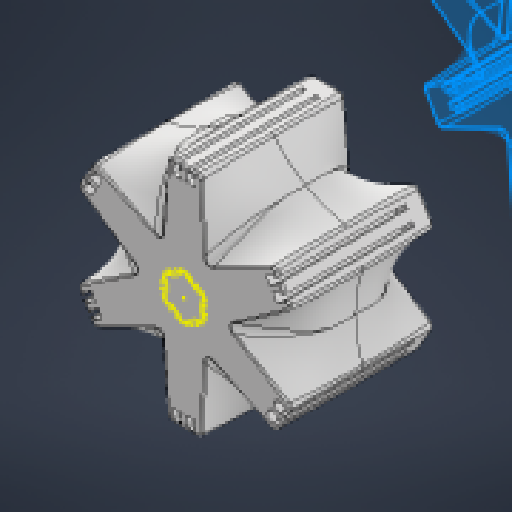
# Autodesk Inventor part: 3DPRINT,HUB
Saved by Autodesk Inventor 2026.1 (Build 301233020, 233B)
## iProperties
Created: 2026-02-05
Part Number: 3DPRINT,HUB
Material: Generic
Document SubType Name: Modeling
Designer: Owen L
Density: 1 g/cm^3
Appearance: Default
Mass: 1846.51 g
Surface Area: 1357.43 cm^2
Volume: 1846.51 cm^3
Author: Owen L
Autodesk Inventor part; units mm, degrees
ref_plane "YZ Plane" through (0, 0, 0) normal (1, 0, 0) x (0, 1, 0)
ref_plane "XZ Plane" through (0, 0, 0) normal (0, 1, 0) x (-1, 0, 0)
ref_plane "XY Plane" through (0, 0, 0) normal (0, 0, 1) x (1, 0, 0)
sketch "Sketch1" plane through (0, 0, 0) normal (0, 0, 1) x (1, 0, 0)
  line L0 (0, 0) -> (0, 85.725) construction
  line L1 (-12.7, 85.725) -> (12.7, 85.725)
  line L2 (-80.59, 31.864) -> (-67.89, 53.861)
  line L3 (-67.89, -53.861) -> (-80.59, -31.864)
  line L4 (12.7, -85.725) -> (-12.7, -85.725)
  line L5 (80.59, -31.864) -> (67.89, -53.861)
  line L6 (67.89, 53.861) -> (80.59, 31.864)
  arc A0 (12.7, 85.725) -> (67.89, 53.861) centre (81.7917, 141.6674) ccw
  arc A1 (80.59, 31.864) -> (80.59, -31.864) centre (163.5834, 0) ccw
  arc A2 (67.89, -53.861) -> (12.7, -85.725) centre (81.7917, -141.6674) ccw
  arc A3 (-12.7, -85.725) -> (-67.89, -53.861) centre (-81.7917, -141.6674) ccw
  arc A4 (-80.59, -31.864) -> (-80.59, 31.864) centre (-163.5834, 0) ccw
  arc A5 (-67.89, 53.861) -> (-12.7, 85.725) centre (-81.7917, 141.6674) ccw
  dimension "d0" = 85.725
  dimension "d1" = 25.4
  dimension "d4" = 360
  dimension "d6" = 88.9
  constraints: 14 end point, 12 point on circle, 6 centre point, 5 equal radius, 1 horizontal, 1 midpoint, 1 vertical, 19 other
  measures "d0" distance of L0.start L0.end
  measures "d1" distance of L1.start L1.end
  measures "d6" radius of A0
extrude "Extrusion5" add sketch "Sketch1" along normal mid plane 107.95
sketch "Sketch7" plane through (0, 0, 53.975) normal (0, 0, 1) x (1, 0, 0)
  line L0 (-12.7, -85.725) -> (12.7, -85.725) projected
  line L1 (6.6675, -85.725) -> (6.6675, -82.55)
  line L2 (6.6675, -82.55) -> (8.5725, -82.55)
  line L3 (8.5725, -82.55) -> (8.5725, -76.2)
  line L4 (8.5725, -76.2) -> (1.5875, -76.2)
  line L5 (1.5875, -76.2) -> (1.5875, -82.55)
  line L6 (1.5875, -82.55) -> (3.4925, -82.55)
  line L7 (3.4925, -82.55) -> (3.4925, -85.725)
  line L8 (-3.4925, -85.725) -> (-3.4925, -82.55)
  line L9 (-3.4925, -82.55) -> (-1.5875, -82.55)
  line L10 (-1.5875, -82.55) -> (-1.5875, -76.2)
  line L11 (-1.5875, -76.2) -> (-8.5725, -76.2)
  line L12 (-8.5725, -76.2) -> (-8.5725, -82.55)
  line L13 (-8.5725, -82.55) -> (-6.6675, -82.55)
  line L14 (-6.6675, -82.55) -> (-6.6675, -85.725)
  line L15 (0, -85.725) -> (0, 0) construction
  dimension "d73" = 6.35
  dimension "d74" = 1.905
  dimension "d75" = 3.175
  dimension "d76" = 3.175
  dimension "d77" = 1.5875
  constraints: 30 end point, 10 perpendicular, 8 point on line, 6 equal length, 3 vertical, 1 midpoint, 1 other
  measures "d73" distance of L2.end L3.end
  measures "d74" distance of L1.end L2.end
  measures "d75" distance between parallel lines of L7 L1
  measures "d76" distance of L1.start L1.end
  measures "d77" distance between parallel lines of L15 L5
extrude "Extrusion6" cut sketch "Sketch7" against normal blind 95.25
pattern_circular "Circular Pattern3" count 6 over 360 about axis through (0, 0, -10) along (0, 0, 1) of "Extrusion6"
body "Solid3"
